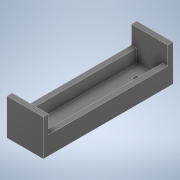
# Autodesk Inventor part: batteryBox
Saved by Autodesk Inventor 2022 (Build 260153000, 153)
## iProperties
Created: 2021-07-08
Part Number: batteryBox
Material: アセタール樹脂、黒
Document SubType Name: Modeling
Designer: ken
Density: 1.425 g/cm^3
Appearance: 滑らか - 黒
Author: ken
Autodesk Inventor part; units mm, degrees
ref_plane "YZ Plane" through (0, 0, 0) normal (1, 0, 0) x (0, 1, 0)
ref_plane "XZ Plane" through (0, 0, 0) normal (0, 1, 0) x (-1, 0, 0)
ref_plane "XY Plane" through (0, 0, 0) normal (0, 0, 1) x (1, 0, 0)
sketch "スケッチ1" plane through (0, 0, 0) normal (0, 1, 0) x (-1, 0, 0)
  line L0 (0, 0) -> (21, 0)
  line L1 (21, 0) -> (21, -75)
  line L2 (21, -75) -> (0, -75)
  line L3 (0, -75) -> (0, 0)
  dimension "d0" = 21
  dimension "d3" = 75
  constraints: 8 end point, 2 parallel, 1 horizontal, 1 perpendicular
  measures "d0" distance of L1.end L2.end
  measures "d3" distance between parallel lines of L2 L0
extrude "押し出し1" add sketch "スケッチ1" along normal blind 3
sketch "スケッチ2" plane through (0, 3, 0) normal (0, 1, 0) x (1, 0, 0)
  line L0 (-21, 0) -> (0, 0) projected
  line L1 (0, 75) -> (-21, 75) projected
  line L2 (-21, 75) -> (-21, 0) projected
  point P0 (-10.5, 10.65)
  point P1 (-10.5, 64.35)
  dimension "d4" = 53.7
  dimension "d5" = 10.65
  dimension "d7" = 10.5
  constraints: 1 vertical alignment
  measures "d4" distance of point (-10.5, 64.35) point (-10.5, 10.65)
  measures "d5" distance from line of L0 point (-10.5, 10.65)
  measures "d7" distance from line of L2 point (-10.5, 10.65)
hole "穴1" at (-10.5, 3, -10.65) at (-10.5, 3, -64.35) direction (0, -1, 0) diameter 3.2 end through all
sketch "スケッチ3" plane through (0, 3, 0) normal (0, 1, 0) x (1, 0, 0)
  line L0 (0, 75) -> (-21, 75) projected
  line L1 (-21, 0) -> (0, 0) projected
  line L2 (-21, 75) -> (0, 75)
  line L3 (0, 75) -> (0, 0)
  line L4 (0, 0) -> (-21, 0)
  line L5 (-21, 0) -> (-21, 75)
  line L6 (-18, 72) -> (-3, 72)
  line L7 (-3, 72) -> (-3, 3)
  line L8 (-3, 3) -> (-18, 3)
  line L9 (-18, 3) -> (-18, 72)
  dimension "d15" = 3
  dimension "d16" = 3
  dimension "d17" = 3
  dimension "d18" = 3
  constraints: 16 end point, 4 parallel, 2 horizontal, 2 perpendicular
  measures "d15" distance between parallel lines of L0 L6
  measures "d16" distance between parallel lines of L1 L8
  measures "d17" distance between parallel lines of L3 L7
  measures "d18" distance between parallel lines of L5 L9
extrude "押し出し2" add sketch "スケッチ3" along normal blind 7.5
sketch "スケッチ4" plane through (0, 10.5, 0) normal (0, 1, 0) x (1, 0, 0)
  line L0 (0, 75) -> (-21, 75) projected
  line L1 (0, 0) -> (0, 75) projected
  line L2 (-21, 75) -> (0, 75)
  line L3 (0, 75) -> (0, 72)
  line L4 (0, 72) -> (-21, 72)
  line L5 (-21, 72) -> (-21, 75)
  line L6 (-21, 75) -> (-21, 0) projected
  line L7 (-21, 0) -> (0, 0)
  line L8 (0, 0) -> (0, 3)
  line L9 (0, 3) -> (-21, 3)
  line L10 (-21, 3) -> (-21, 0)
  dimension "d21" = 3
  dimension "d22" = 3
  constraints: 16 end point, 4 parallel, 2 horizontal, 2 perpendicular, 2 point on line
  measures "d21" distance of L2.end L3.end
  measures "d22" distance of L8.end L7.end
extrude "押し出し3" add sketch "スケッチ4" along normal blind 10.5 contours L1 L4 L5 L0 | L1 L7 L6 L9
